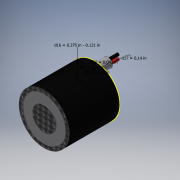
# Autodesk Inventor part: CE-075-12C
Saved by Autodesk Inventor 2018.2 (Build 222227000, 227)
## iProperties
Created: 2015-07-27
Material: Generic
Vendor: AEC MAGNETICS
Document SubType Name: Modeling
Designer: ARNOLDJ
Density: 1 g/cm^3
Appearance: Default
Description: 12VDC CIRCULAR ELECTROMAGNET
Part Number: CE-075-12C
RuleStatus: InUse
AfterDocSave0: file://Part Number Cleaner
DESIGN DEPARTMENT: HHMI: JRC - ID&F
ALTERED ITEM PART NUMBER: N/A
ALTERED ITEM VENDOR: N/A
ALTERED ITEM DESCRIPTION: N/A
Author: ARNOLDJ
Revision Number: 0
Autodesk Inventor part; units mm, degrees
ref_plane "YZ Plane" through (0, 0, 0) normal (1, 0, 0) x (0, 1, 0)
ref_plane "XZ Plane" through (0, 0, 0) normal (0, 1, 0) x (-1, 0, 0)
ref_plane "XY Plane" through (0, 0, 0) normal (0, 0, 1) x (1, 0, 0)
sketch "Sketch1" plane through (0, 0, 0) normal (0, 0, 1) x (1, 0, 0)
  circle A0 centre (0, 0) radius 9.525
  dimension "d0" = 19.05
  constraints: 1 centre point, 1 coincident
  measures "d0" diameter of A0
extrude "Extrusion1" add sketch "Sketch1" along normal blind 19.05
sketch "Sketch2" plane through (0, 0, 19.05) normal (0, 0, 1) x (1, 0, 0)
  circle A0 centre (0, 0) radius 8.1534
  circle A1 centre (0, 0) radius 4.445
  circle A2 centre (0, 0) radius 9.525 projected
  dimension "d3" = 8.89
  dimension "d4" = 1.3716
  constraints: 2 centre point, 2 coincident
  measures "d3" diameter of A1
  measures "d4" radial gap between concentric circles of A0 A2
extrude "Extrusion2" cut sketch "Sketch2" against normal blind 0.254 contours A0
hole "Hole1" at (0, 0, 0) direction (0, 0, 1) diameter 2.6416 depth 7.9375 tip angle 118 thread size "6-32 UNC" class "2B" standard "ANSI Unified Screw Threads"
sketch "Sketch3" plane through (0, 0, 0) normal (0, 0, -1) x (-1, 0, 0)
  circle A0 centre (0, 6.4516) radius 1.778
  circle A1 centre (0, 0) radius 9.525 projected
  circle A2 centre (0, 7.2136) radius 0.5461
  circle A3 centre (0, 5.6896) radius 0.5461
  dimension "d16" = 6.4516
  dimension "d17" = 3.556
  dimension "d20" = 1.0922
  dimension "d21" = 0.762
  dimension "d22" = 0.762
  constraints: 3 centre point, 1 equal radius
  measures "d16" distance of A0.centre A1.centre
  measures "d17" diameter of A0
  measures "d20" diameter of A2
  measures "d21" distance of A2.centre A0.centre
  measures "d22" distance of A0.centre A3.centre
extrude "Extrusion3" add sketch "Sketch3" along normal blind 5.08 contours A0 | A2 | A3
sketch "Sketch4" plane through (0, 6.4516, -5.08) normal (0, 0, -1) x (-1, 0, 0)
  circle A0 centre (0, 0.773) radius 0.5212
  circle A1 centre (0, -0.7642) radius 0.5469
  point P0 (0, -6.4516)
  constraints: 2 centre point
extrude "Extrusion4" add sketch "Sketch4" along normal blind 3.81
body "Solid1"
